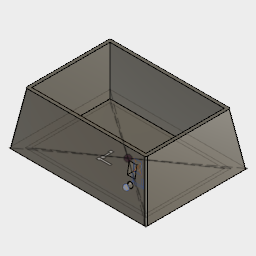
Jenkins_Monitor_Base v1 (Autodesk Fusion 360 design; units mm, degrees)
Autodesk Fusion 360 part; units mm, degrees
sketch "Sketch1" plane through (0, 0, 0) normal (0, 0, 1) x (1, 0, 0)
  line L0 (-70, 48) -> (70, 48)
  line L1 (70, 48) -> (70, -48)
  line L2 (70, -48) -> (-70, -48)
  line L3 (-70, -48) -> (-70, 48)
  line L4 (-70, 48) -> (70, -48) construction
  line L5 (70, 48) -> (-70, -48) construction
  line L6 (-74, 52) -> (74, 52)
  line L7 (74, 52) -> (74, -52)
  line L8 (74, -52) -> (-74, -52)
  line L9 (-74, -52) -> (-74, 52)
  line L10 (-74, 52) -> (74, -52) construction
  line L11 (74, 52) -> (-74, -52) construction
  line L12 (-84, 62) -> (84, 62)
  line L13 (84, 62) -> (84, -62)
  line L14 (84, -62) -> (-84, -62)
  line L15 (-84, -62) -> (-84, 62)
  line L16 (-84, 62) -> (84, -62) construction
  line L17 (84, 62) -> (-84, -62) construction
  dimension "d1" = 140
  dimension "d2" = 96
  dimension "d3" = 148
  dimension "d4" = 104
  dimension "d9" = 168
  dimension "d10" = 124
  measures "d1" distance of L1.end L2.end
  measures "d2" distance of L0.end L1.end
  measures "d3" distance of L7.end L8.end
  measures "d4" distance of L6.end L7.end
  measures "d9" distance of L13.end L14.end
  measures "d10" distance of L12.end L13.end
extrude "Extrude1" add sketch "Sketch1" along normal blind 4 contours L0 L1 L2 L3
extrude "Extrude2" add sketch "Sketch1" along normal blind 64 contours L6 L7 L8 L9
ref_plane "WorkPlane1" through (0, 0, 64) normal (0, 0, 1) x (1, 0, 0)
sketch "Sketch2" plane through (0, 0, 64) normal (0, 0, 1) x (1, 0, 0)
  line L0 (-74, 52) -> (74, 52)
  line L1 (74, 52) -> (74, -52)
  line L2 (74, -52) -> (-74, -52)
  line L3 (-74, -52) -> (-74, 52)
  line L4 (-74, 52) -> (74, -52) construction
  line L5 (74, 52) -> (-74, -52) construction
  point P0 (-74, 52)
loft "Loft1" add profiles "Sketch1", "Sketch2" section 1 contours L12 L13 L14 L15 section 2
extrude "Extrude3" cut sketch "Sketch1" along normal up to surface (64 mm away) contours L0 L1 L2 L3
extrude "Extrude4" add sketch "Sketch1" along normal blind 4 contours L0 L1 L2 L3
ref_plane "WorkPlane2" through (0, -62, 0) normal (0, 1, 0) x (0, 0, 1)
sketch "Sketch3" plane through (0, -62, 0) normal (0, 1, 0) x (1, 0, 0)
  circle A0 centre (60, -30) radius 3
  dimension "d17" = 6
  measures "d17" diameter of A0
extrude "Extrude5" cut sketch "Sketch3" along normal up to surface (14 mm away)
ref_plane "WorkPlane3" through (0, -48, 34) normal (0, 1, 0) x (-1, 0, 0)
sketch "Sketch4" plane through (0, -48, 34) normal (0, 1, 0) x (1, 0, 0)
  line L0 (67, 7.4) -> (53, 7.4)
  line L1 (53, 7.4) -> (53, 9.4)
  line L2 (53, 9.4) -> (67, 9.4)
  line L3 (67, 9.4) -> (67, 7.4)
  line L4 (67, 7.4) -> (65, 7.4)
  line L5 (65, 7.4) -> (65, -0.6)
  line L6 (65, -0.6) -> (67, -0.6)
  line L7 (67, -0.6) -> (67, 7.4)
  line L8 (53, 7.4) -> (55, 7.4)
  line L9 (55, 7.4) -> (55, -0.6)
  line L10 (55, -0.6) -> (53, -0.6)
  line L11 (53, -0.6) -> (53, 7.4)
  dimension "d21" = 14
  dimension "d22" = 2
  dimension "d23" = 8
  dimension "d24" = 2
  dimension "d25" = 8
  measures "d21" distance of L0.start L0.end
  measures "d22" distance of L0.start L2.end
  measures "d23" distance of L0.start L6.end
  measures "d24" distance of L0.end L8.end
  measures "d25" distance of L0.end L10.end
extrude "Extrude6" add sketch "Sketch4" along normal blind 28
sketch "Sketch5" plane through (0, -48, 0) normal (0, 1, 0) x (-1, 0, 0)
  line L0 (-65, 26.6) -> (-55, 26.6)
  line L1 (-55, 26.6) -> (-55, 34.6)
  line L2 (-55, 34.6) -> (-53, 34.6)
  line L3 (-53, 34.6) -> (-53, 24.6)
  line L4 (-53, 24.6) -> (-67, 24.6)
  line L5 (-67, 24.6) -> (-67, 34.6)
  line L6 (-67, 34.6) -> (-65, 34.6)
  line L7 (-65, 34.6) -> (-65, 26.6)
  circle A0 centre (-60, 30) radius 3
  line L8 (-70, 4) -> (70, 4)
  line L9 (70, 4) -> (70, 64)
  line L10 (70, 64) -> (-70, 64)
  line L11 (-70, 64) -> (-70, 4)
  line L12 (-55.3, 38) -> (-64.7, 38)
  line L13 (-64.7, 38) -> (-64.7, 52)
  line L14 (-64.7, 52) -> (-55.3, 52)
  line L15 (-55.3, 52) -> (-55.3, 38)
  line L16 (-55.3, 38) -> (-64.7, 52) construction
  line L17 (-64.7, 38) -> (-55.3, 52) construction
  point P0 (-60, 45)
  dimension "d28" = 14
  dimension "d29" = 9.4
  measures "d28" distance of L12.end L13.end
  measures "d29" distance of L13.end L14.end
extrude "Extrude7" cut sketch "Sketch5" along normal up to surface contours L12 L13 L14 L15 end surface at (-33.6547, -57.1282, 31.1794)
fillet "Fillet1" radius 2 4 edges at (79, -57, 32) (79, 57, 32) (-79, 57, 32) (-79, -57, 32)
chamfer "Chamfer1" distance 0.4 angle 45 2 edges at (55, -34, 34.6) (65, -34, 34.6)
fillet "Fillet2" radius 0.4 1 edges at (57.203, -48, 28.9152)
fillet "Fillet3" radius 0.4 1 edges at (60, -56.8438, 33)
